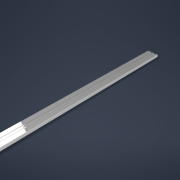
# Autodesk Inventor part: Rail_TypeB
Saved by Autodesk Inventor 2021.2 (Build 252289000, 289)
## iProperties
Created: 2021-06-16
Part Number: Rail_TypeB
Material: Aluminum
Document SubType Name: Modeling
Designer: joanh
Density: 2.7 g/cm^3
Appearance: Aluminum - Polished
Author: joanh
Autodesk Inventor part; units mm, degrees
ref_plane "YZ Plane" through (0, 0, 0) normal (1, 0, 0) x (0, 1, 0)
ref_plane "XZ Plane" through (0, 0, 0) normal (0, 1, 0) x (-1, 0, 0)
ref_plane "XY Plane" through (0, 0, 0) normal (0, 0, 1) x (1, 0, 0)
sketch "Rail_TypeB_Sketch" plane through (0, 0, 0) normal (0, 0, 1) x (1, 0, 0)
  line L0 (-11, 3.75) -> (-1.6, 3.75)
  line L1 (16.5, 3.75) -> (16.5, -3.75)
  line L2 (16.5, -3.75) -> (13.2, -3.75)
  line L3 (-11, -3.75) -> (-11, -1.6)
  arc A0 (-1.9596, 2.25) -> (-1.9596, 0.25) centre (0, 1.25) ccw construction
  line L4 (-11, 0) -> (16.5, 0) construction
  line L5 (0, 3.75) -> (0, -3.75) construction
  line L6 (-11, 1.6) -> (-9.5, 1.6)
  line L7 (-5, 1.6) -> (-5, -1.6)
  line L8 (-5, -1.6) -> (-7, -1.6)
  line L9 (-11, 1.6) -> (-11, 3.75)
  line L10 (-11, -1.6) -> (-11, 1.6) construction
  line L11 (-7, 2.95) -> (-9.5, 2.95)
  line L12 (-9.5, 2.95) -> (-9.5, 1.6)
  line L13 (-9.5, -2.95) -> (-7, -2.95)
  line L14 (-7, -2.95) -> (-7, -1.6)
  line L15 (-9.5, 1.6) -> (-7, 1.6) construction
  line L16 (-7, 1.6) -> (-5, 1.6)
  line L17 (-9.5, -1.6) -> (-11, -1.6)
  line L18 (-7, -1.6) -> (-9.5, -1.6) construction
  line L19 (-7, -1.6) -> (-7, 1.6) construction
  line L20 (-9.5, -1.6) -> (-9.5, -2.95)
  line L21 (-9.5, 1.6) -> (-9.5, -1.6) construction
  line L22 (-7, 1.6) -> (-7, 2.95)
  line L23 (-6, -3.75) -> (-6, -3.25)
  line L24 (-6, -3.25) -> (4, -3.25)
  line L25 (4, -3.25) -> (4, -3.75)
  line L26 (-6, -3.75) -> (-11, -3.75)
  line L27 (4, -3.75) -> (-6, -3.75) construction
  line L28 (1.6, -1.25) -> (-1.6, -1.25)
  line L29 (-1.6, -1.25) -> (-1.6, -0.26)
  line L30 (1.6, 3.75) -> (1.6, 2.76)
  line L31 (1.6, -1.25) -> (-1.6, 3.75) construction
  line L32 (-1.6, -1.25) -> (1.6, 3.75) construction
  line L33 (-3, 2.25) -> (-1.9596, 2.25)
  line L34 (3, 2.25) -> (3, 0.25)
  line L35 (3, 0.25) -> (1.9596, 0.25)
  line L36 (-3, 0.25) -> (-3, 2.25)
  line L37 (-3, 2.25) -> (3, 0.25) construction
  line L38 (3, 2.25) -> (-3, 0.25) construction
  arc A1 (-1.6, 2.76) -> (-1.9596, 2.25) centre (0, 1.25) ccw
  arc A2 (1.9596, 2.25) -> (1.6, 2.76) centre (0, 1.25) ccw
  arc A3 (1.6, 2.76) -> (-1.6, 2.76) centre (0, 1.25) ccw construction
  arc A4 (1.9596, 0.25) -> (1.9596, 2.25) centre (0, 1.25) ccw construction
  arc A5 (1.6, -0.26) -> (1.9596, 0.25) centre (0, 1.25) ccw
  arc A6 (-1.6, -0.26) -> (1.6, -0.26) centre (0, 1.25) ccw construction
  arc A7 (-1.9596, 0.25) -> (-1.6, -0.26) centre (0, 1.25) ccw
  line L39 (-1.9596, 2.25) -> (1.9596, 2.25) construction
  line L40 (-1.9596, 0.25) -> (-3, 0.25)
  line L41 (1.9596, 2.25) -> (3, 2.25)
  line L42 (1.9596, 0.25) -> (-1.9596, 0.25) construction
  line L43 (-1.6, 2.76) -> (-1.6, 3.75)
  line L44 (1.6, 2.76) -> (1.6, -0.26) construction
  line L45 (1.6, -0.26) -> (1.6, -1.25)
  line L46 (-1.6, -0.26) -> (-1.6, 2.76) construction
  line L47 (10, 3.75) -> (10, -3.75) construction
  line L48 (5.2, 3.75) -> (5.2, 2.25)
  line L49 (5.2, 2.25) -> (14.8, 2.25)
  line L50 (14.8, 2.25) -> (14.8, 3.75)
  line L51 (5.2, 3.75) -> (14.8, 3.75) construction
  line L52 (14.8, 3.75) -> (16.5, 3.75)
  line L53 (13.2, -3.75) -> (13.2, -2.25)
  line L54 (13.2, -2.25) -> (14.8, -2.25)
  line L55 (14.8, -2.25) -> (14.8, 0.25)
  line L56 (14.8, 0.25) -> (5.2, 0.25)
  line L57 (5.2, 0.25) -> (5.2, -2.25)
  line L58 (5.2, -2.25) -> (6.8, -2.25)
  line L59 (6.8, -2.25) -> (6.8, -3.75)
  line L60 (6.8, -3.75) -> (4, -3.75)
  line L61 (13.2, -3.75) -> (6.8, -3.75) construction
  line L62 (-1.6, 3.75) -> (0, 3.75) construction
  line L63 (0, 3.75) -> (1.6, 3.75) construction
  line L64 (1.6, 3.75) -> (5.2, 3.75)
  point P0 (0, 0)
  dimension "d0" = 27.5
  dimension "d1" = 7.5
  dimension "d3" = 3.75
  dimension "d5" = 4.4
  dimension "d6" = 2.5
  dimension "d8" = 16.5
  dimension "d9" = 6
  dimension "d10" = 3.2
  dimension "d11" = 1.6
  dimension "d12" = 11
  dimension "d13" = 1.5
  dimension "d14" = 4
  dimension "d15" = 5.9
  dimension "d16" = 2.95
  dimension "d17" = 0.5
  dimension "d18" = 10
  dimension "d19" = 5
  dimension "d20" = 3.2
  dimension "d21" = 5
  dimension "d22" = 6
  dimension "d23" = 2
  dimension "d24" = 10
  dimension "d25" = 9.6
  dimension "d26" = 4.8
  dimension "d27" = 6
  dimension "d28" = 1.5
  dimension "d29" = 4
  dimension "d30" = 6.4
  dimension "d31" = 3.2
  dimension "d32" = 9.6
  dimension "d33" = 4.8
  constraints: 130 end point, 49 perpendicular, 47 parallel, 16 point on circle, 11 horizontal, 11 point on line, 9 midpoint, 8 centre point, 3 vertical
  measures "d0" distance of L1.end L3.start
  measures "d1" distance of L1.start L1.end
  measures "d3" distance from line of L0 point (0, 0)
  measures "d5" diameter of A0
  measures "d6" distance from line of A0.centre L0
  measures "d8" distance from line of L1 A0.centre
  measures "d9" distance of L6.start L7.start
  measures "d10" distance of L7.start L7.end
  measures "d11" distance between parallel lines of L4 L6
  measures "d12" distance between parallel lines of L5 L9
  measures "d13" distance between parallel lines of L9 L12
  measures "d14" distance between parallel lines of L14 L9
  measures "d15" distance between parallel lines of L13 L11
  measures "d16" distance between parallel lines of L4 L11
  measures "d17" distance of L23.start L23.end
  measures "d18" distance of L23.end L24.end
  measures "d19" distance between parallel lines of L3 L23
  measures "d20" distance of L0.end L30.start
  measures "d21" distance of L28.end L0.end
  measures "d22" distance of L34.end L36.start
  measures "d23" distance of L34.start L34.end
  measures "d24" distance between parallel lines of L5 L47
  measures "d25" distance between parallel lines of L50 L48
  measures "d26" distance between parallel lines of L50 L47
  measures "d27" distance between parallel lines of L2 L49
  measures "d28" distance of L2.end L53.end
  measures "d29" distance between parallel lines of L2 L56
  measures "d30" distance between parallel lines of L53 L59
  measures "d31" distance between parallel lines of L47 L53
  measures "d32" distance between parallel lines of L57 L55
  measures "d33" distance between parallel lines of L47 L57
extrude "Extrusion1" add sketch "Rail_TypeB_Sketch" against normal blind 426.72
fillet "Fillet1_0.5 mm" radius 0.5 5 edges at (-11, 3.75, -213.36) (5.2, 3.75, -213.36) (14.8, 3.75, -213.36) (6.8, -3.75, -213.36) (13.2, -3.75, -213.36)
fillet "Fillet2_0.1 mm" radius 0.1 35 edges at (-1.6, 3.75, -213.36) (1.6, 3.75, -213.36) (5.2, 2.25, -213.36) (14.8, 2.25, -213.36) (16.5, 3.75, -213.36) (16.5, -3.75, -213.36) (13.2, -2.25, -213.36) (14.8, -2.25, -213.36) (14.8, 0.25, -213.36) (5.2, 0.25, -213.36) (5.2, -2.25, -213.36) (6.8, -2.25, -213.36) (4, -3.75, -213.36) (4, -3.25, -213.36) (-6, -3.25, -213.36) (-6, -3.75, -213.36) (-11, -3.75, -213.36) (-11, -1.6, -213.36) (-9.5, -1.6, -213.36) (-9.5, -2.95, -213.36) (-7, -2.95, -213.36) (-7, -1.6, -213.36) (-5, -1.6, -213.36) (-5, 1.6, -213.36) (-7, 1.6, -213.36) (-7, 2.95, -213.36) (-9.5, 2.95, -213.36) (-9.5, 1.6, -213.36) (-11, 1.6, -213.36) (-3, 2.25, -213.36) (-3, 0.25, -213.36) (-1.6, -1.25, -213.36) (1.6, -1.25, -213.36) (3, 0.25, -213.36) (3, 2.25, -213.36)
equation "\"d3\" = 0.5 * d1"
equation "\"d11\" = 0.5 * d10"
equation "\"d16\" = 0.5 * d15"
equation "\"d26\" = 0.5 * d25"
equation "\"d31\" = 0.5 * d30"
equation "\"d32\" = d25"
equation "\"d33\" = 0.5 * d32"
body "Solid1"
